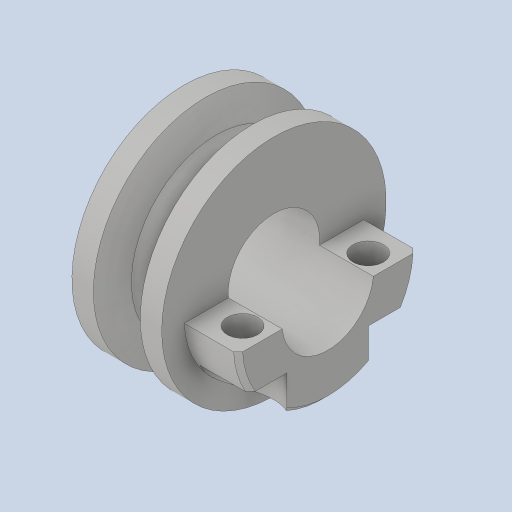
# Autodesk Inventor part: MBRDAC23-2-8_p1
Saved by Autodesk Inventor 2024 (Build 280153000, 153)
## iProperties
Category: PARTsolutions
Company: MISUMI
Created: 2024-03-05
Part Number: MBRDAC23-2-8_p1
Material: Generic
Catalog Web Link: www.cadenas.de
Description: MBRDC, MBRDAC_part1-Pulleys for Round Belts - Clamping Type - Trapezoid Groove
Vendor: MISUMI
Document SubType Name: Modeling
Designer: psAdmin
Manufacturer: MISUMI
Mass: 4.25663 g
Surface Area: 25.1033 cm^2
Volume: 4.25663 cm^3
Density: 1 g/cm^3
Appearance: PSOLRGB-175-175-175
PSOL_IDENT_0: {$CADENAS_DATA/23d-libs/misumi/metric/52_belts_pulleys/mbrdc/mbrdc_part1.prj},201 {VTYP=3D},{NB=MBRD
PSOL_IDENT_1: AC23-2-8_p1},{LINA=MBRDAC23-2-8},{NN=MBRDC, MBRDAC_part1},{DATE=01.02.2024 02:38:37},{GEOMDATE=19.01
PSOL_IDENT_2: .2024 06:52:40},{VERSION=},{LINEID=30},{WBVAR=MAT,PD,DDS,ALT1},{WBNUMERIC=PD,DDS}  {NB=MBRDAC23-2-8_
PSOL_IDENT_3: p1},{LINA=MBRDAC23-2-8},{KT=DUMMY},{PN=MBRDAC23-2-8},{TYPE=MBRDAC},{MAT=2},{ST=Clear Anodizing},{AC=
PSOL_IDENT_4: Hexagon Socket Head Cap Screw (x2) Stainless Steel},{PD=23},{PD0=23,28,30,40,45,48,60,80},{U=2.0},{D
PSOL_IDENT_5: DS=8.00},{DS0=5,6,6.35,8},{D=20},{D1=25},{D2=19},{HH=2.0},{W=4.4},{L=16},{T=10},{LL=2.5},{X=7.0},{Y=
PSOL_IDENT_6: 3.5},{M=M3},{CBD=4},{MM=3.000},{MMMIN=2.459},{DD1=6.5},{DD2=3.5},{ALT1=},{ALT1ALG='','w/o DC (Outer
PSOL_IDENT_7: Diameter Cut)','-DC','with DC (Outer Diameter Cut)'},{DC=0.0}
NB: MBRDAC23-2-8_p1
NN: MBRDC, MBRDAC_part1
NT: Pulleys for Round Belts - Clamping Type - Trapezoid Groove
NBSYN: $PN._p1
LINA: MBRDAC23-2-8
CATALOG: Misumi
PN: MBRDAC23-2-8
TYPE: MBRDAC
MAT: 5052 Aluminum Alloy
ST: Clear Anodizing
AC: Hexagon Socket Head Cap Screw (x2) Stainless Steel
PD: 23
U: 2
DDS: 8
D: 20
D1: 25
D2: 19
HH: 2
W: 4.4
L: 16
T: 10
LL: 2.5
X: 7
Y: 3.5
M: M3
CBD: 4
DD1: 6.5
DD2: 3.5
ALT1: w/o DC (Outer Diameter Cut)
DC: 0
SUPPLIER: MISUMI
ARTICLENO: MBRDAC23-2-8_p1
BOMINFO: MBRDAC23-2-8
CREATOR: CADENAS GmbH
Title: MBRDAC23-2-8
Author: Cadenas PARTsolutions
Comments: Pulleys for Round Belts - Clamping Type - Trapezoid Groove
Autodesk Inventor part; units mm, degrees
sketch "Sketch_1" plane through (0, 0, 0) normal (0, 0, 1) x (1, 0, 0)
  line L0 (5, 0) -> (-5, 0)
  line L1 (-5, 0) -> (-5, 12.5)
  line L2 (-5, 12.5) -> (-2.6142, 12.5)
  line L3 (-2.6142, 12.5) -> (-1.3716, 9.5)
  line L4 (-1.3716, 9.5) -> (1.3716, 9.5)
  line L5 (1.3716, 9.5) -> (2.6142, 12.5)
  line L6 (2.6142, 12.5) -> (5, 12.5)
  line L7 (5, 12.5) -> (5, 0)
  line L8 (5, 0) -> (-5, 0)
  constraints: 18 end point
revolve "Revolution1" add sketch "Sketch_1" angle 360 about axis through (5, 0, 0) along (1, 0, 0)
sketch "Sketch_2" plane through (0, 0, 0) normal (0, 0, 1) x (1, 0, 0)
  line L0 (5, 0) -> (11, 0)
  line L1 (11, 0) -> (11, -9.5)
  line L2 (11, -9.5) -> (10.5, -10)
  line L3 (10.5, -10) -> (5, -10)
  line L4 (5, -10) -> (5, 0)
  line L5 (5, 0) -> (11, 0)
  constraints: 12 end point
revolve "Revolution2" add sketch "Sketch_2" angle 180 mid plane about axis through (5, 0, 0) along (1, 0, 0)
sketch "Sketch_3" plane through (0, 0, 0) normal (0, 0, 1) x (1, 0, 0)
  line L0 (5, -0.5) -> (11, -0.5)
  line L1 (11, -0.5) -> (11, 0)
  line L2 (11, 0) -> (5, 0)
  line L3 (5, 0) -> (5, -0.5)
  constraints: 8 end point
extrude "Extrusion1" cut sketch "Sketch_3" along normal mid plane 40
sketch "Sketch_9" plane through (8.5, 0, 0) normal (1, 0, 0) x (0, 0, -1)
  line L0 (7, -10) -> (7, -0.5)
  line L1 (7, -0.5) -> (8.5, -0.5)
  line L2 (8.5, -0.5) -> (8.2295, -0.7705)
  line L3 (8.2295, -0.7705) -> (8.2295, -9.7295)
  line L4 (8.2295, -9.7295) -> (8.5, -10)
  line L5 (8.5, -10) -> (7, -10)
  line L6 (7, -10) -> (7, -0.5)
  constraints: 14 end point
revolve "Revolution4" cut sketch "Sketch_9" angle 360 about axis through (8.5, -10, -7) along (0, -1, 0)
sketch "Sketch_6" plane through (8.5, 0, 0) normal (1, 0, 0) x (0, 0, -1)
  line L0 (-7, -10) -> (-7, -0.5)
  line L1 (-7, -0.5) -> (-5.5, -0.5)
  line L2 (-5.5, -0.5) -> (-5.7705, -0.7705)
  line L3 (-5.7705, -0.7705) -> (-5.7705, -9.7295)
  line L4 (-5.7705, -9.7295) -> (-5.5, -10)
  line L5 (-5.5, -10) -> (-7, -10)
  line L6 (-7, -10) -> (-7, -0.5)
  constraints: 14 end point
revolve "Revolution5" cut sketch "Sketch_6" angle 360 about axis through (8.5, -10, 7) along (0, -1, 0)
ref_plane "part1_to_part2_XY" through (5, 0, 0) normal (1, 0, 0) x (0, 0, -1)
ref_plane "part1_to_part2_YZ" through (5, 0, 0) normal (0, 0, -1) x (0, 1, 0)
ref_plane "part1_to_part2_ZX" through (5, 0, 0) normal (0, 1, 0) x (1, 0, 0)
sketch "スケッチ7" plane through (-5, 0, 0) normal (-1, 0, 0) x (0, 0, 1)
  circle A0 centre (0, 0) radius 5.1
  dimension "d12" = 10.2
  constraints: 1 centre point, 1 coincident
  measures "d12" diameter of A0
extrude "押し出し2" cut sketch "スケッチ7" against normal through all
ref_plane "作業平面4" through (7.75, -10, 0) normal (0, 1, 0) x (-1, 0, 0)
sketch "スケッチ8" plane through (7.75, -10, 0) normal (0, 1, 0) x (-1, 0, 0)
  circle A0 centre (-0.75, 7) radius 1.2295 projected
  circle A1 centre (-0.75, 7) radius 1.7
  circle A2 centre (-0.75, -7) radius 1.5 projected
  circle A3 centre (-0.75, -7) radius 1.7
  circle A4 centre (-0.75, 7) radius 3.5
  circle A5 centre (-0.75, -7) radius 3.5
  point P0 (7.75, 0)
  dimension "d15" = 3.4
  dimension "d16" = 3.4
  dimension "d17" = 7
  dimension "d18" = 7
  constraints: 4 centre point, 4 coincident
  measures "d15" diameter of A1
  measures "d16" diameter of A3
  measures "d17" diameter of A4
  measures "d18" diameter of A5
extrude "押し出し3" cut sketch "スケッチ8" along normal through all contours A0 | A1 | A2 | A3
extrude "押し出し4" cut sketch "スケッチ8" along normal blind 5 contours A0 | A1 | A2 | A3 | A4 | A5
body "Solid1"
